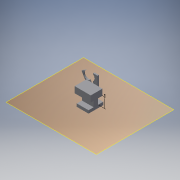
# Autodesk Inventor part: BSF_ShuttleFeeder
Saved by Autodesk Inventor 2018 (Build 220112000, 112)
## iProperties
Created: 2019-03-24
Part Number: BSF_ShuttleFeeder
Material: Generic
Document SubType Name: Modeling
Designer: simon
Density: 1 g/cm^3
Appearance: Default
Author: simon
Autodesk Inventor part; units mm, degrees
ref_plane "YZ Plane" through (0, 0, 0) normal (1, 0, 0) x (0, 1, 0)
ref_plane "XZ Plane" through (0, 0, 0) normal (0, 1, 0) x (-1, 0, 0)
ref_plane "Work Plane1" through (0, 0, 0) normal (0, 0, 1) x (1, 0, 0)
ref_plane "Work Plane2" through (-162, -84, 44) normal (0, 0, 1) x (1, 0, 0)
sketch "Sketch1" plane through (0, 0, 0) normal (0, 0, 1) x (1, 0, 0)
  line L0 (-280, 0) -> (-160, 0) projected
  line L1 (-280, 0) -> (-280, -40) projected
  line L2 (-162, -40) -> (-280, -40) projected
  line L3 (-118, -40) -> (-162, -40) projected
  line L4 (0, -40) -> (-118, -40) projected
  line L5 (0, 0) -> (0, -40) projected
  line L6 (-120, 0) -> (0, 0) projected
  line L7 (-120, 0) -> (-120, 160) projected
  line L8 (0, 160) -> (-120, 160) projected
  line L9 (0, 160) -> (0, 200) projected
  line L10 (-280, 200) -> (0, 200) projected
  line L11 (-280, 160) -> (-280, 200) projected
  line L12 (-160, 160) -> (-280, 160) projected
  line L13 (-160, 0) -> (-160, 160) projected
  line L14 (-160, 87.5) -> (-120, 87.5)
  line L15 (-120, 87.5) -> (-120, 72.5)
  line L16 (-120, 72.5) -> (-160, 72.5)
  line L17 (-160, 72.5) -> (-160, 87.5)
  line L18 (-160, 87.5) -> (-120, 72.5) construction
  line L19 (-120, 87.5) -> (-160, 72.5) construction
  point P0 (-140, 80)
  dimension "d0" = 40
  dimension "d1" = 15
  constraints: 12 end point, 2 midpoint, 2 parallel, 1 horizontal, 1 perpendicular
  measures "d0" distance of L15.end L16.end
  measures "d1" distance of L14.end L15.end
extrude "Extrusion1" add sketch "Sketch1" along normal up to surface (44 mm away) contours L13 L14 L7 L16
ref_plane "Work Plane3" through (0, 0, 0) normal (0, 0, 1) x (1, 0, 0)
sketch "Sketch2" plane through (0, 0, 0) normal (0, 0, 1) x (1, 0, 0)
  line L0 (-120, 87.5) -> (-120, 72.5) projected
  line L1 (-160, 87.5) -> (-120, 87.5) projected
  line L2 (-160, 72.5) -> (-160, 87.5) projected
  line L3 (-120, 72.5) -> (-160, 72.5) projected
  line L4 (-160, 105) -> (-120, 105)
  line L5 (-120, 105) -> (-120, 55)
  line L6 (-120, 55) -> (-160, 55)
  line L7 (-160, 55) -> (-160, 105)
  line L8 (-160, 105) -> (-120, 55) construction
  line L9 (-120, 105) -> (-160, 55) construction
  point P0 (0, 0)
  point P1 (-140, 80)
  dimension "d7" = 40
  dimension "d8" = 50
  constraints: 12 end point, 2 midpoint, 2 parallel, 1 horizontal, 1 perpendicular
  measures "d7" distance of L5.end L6.end
  measures "d8" distance of L4.end L5.end
extrude "Extrusion2" add sketch "Sketch2" along normal blind 10 contours L1 L7 L4 L5 | L5 L6 L7 L3
sketch "Sketch3" plane through (-160, 87.5, 44) normal (0, 1, 0) x (1, 0, 0)
  line L0 (0, 0) -> (55, 0)
  line L1 (55, 0) -> (55, -21)
  line L2 (55, -21) -> (0, -21)
  line L3 (0, -21) -> (0, 0)
  point P0 (160, 44)
  dimension "d11" = 55
  dimension "d12" = 21
  constraints: 8 end point, 2 parallel, 1 horizontal, 1 perpendicular
  measures "d11" distance of L1.end L2.end
  measures "d12" distance of L0.end L1.end
extrude "Extrusion3" add sketch "Sketch3" against normal blind 40
sketch "Sketch4" plane through (-160, 87.5, 10) normal (0, 1, 0) x (1, 0, 0)
  line L0 (40, 0) -> (0, 0) projected
  line L1 (0, 0) -> (0, -55) projected
  line L2 (55, -55) -> (0, -55) projected
  line L3 (55, -34) -> (55, -55) projected
  line L4 (40, -34) -> (55, -34) projected
  line L5 (40, 0) -> (40, -34) projected
  line L6 (55, -55) -> (0, -55) projected
  line L7 (55, -34) -> (0, -34)
  line L8 (0, -34) -> (0, -55)
  line L9 (0, -55) -> (55, -55)
  line L10 (55, -55) -> (55, -34)
  line L11 (0, -44.5) -> (15, -44.5)
  line L12 (0, -44.5) -> (15, -44.5) construction
  circle A0 centre (15, -44.5) radius 4
  point P0 (160, 10)
  dimension "d15" = 15
  dimension "d16" = 0
  dimension "d17" = 8
  constraints: 12 end point, 3 horizontal, 2 parallel, 1 centre point, 1 coincident, 1 collinear, 1 midpoint, 1 perpendicular
  measures "d15" distance of L11.start L11.end
  measures "d16" distance between parallel lines of L11 L12
  measures "d17" diameter of A0
extrude "Extrusion4" add sketch "Sketch4" along normal blind 8 contours A0
sketch "Sketch5" plane through (-160, 87.5, 10) normal (0, 1, 0) x (1, 0, 0)
  circle A0 centre (15, -44.5) radius 4 projected
  line L0 (40, 0) -> (0, 0) projected
  line L1 (0, 0) -> (0, -55) projected
  line L2 (55, -55) -> (0, -55) projected
  line L3 (55, -34) -> (55, -55) projected
  line L4 (40, -34) -> (55, -34) projected
  line L5 (40, 0) -> (40, -34) projected
  circle A1 centre (15, -44.5) radius 4 projected
  line L6 (15, -44.5) -> (28, -44.5)
  line L7 (15, -44.5) -> (28, -44.5) construction
  line L8 (15, -44.5) -> (2, -44.5)
  line L9 (15, -44.5) -> (28, -44.5) construction
  line L10 (28, -44.5) -> (38, -44.5)
  line L11 (38, -44.5) -> (38, -84.5)
  line L12 (38, -84.5) -> (28, -84.5)
  line L13 (28, -84.5) -> (28, -44.5)
  line L14 (28, -44.5) -> (23, -44.5)
  line L15 (23, -44.5) -> (23, -84.5)
  line L16 (23, -84.5) -> (28, -84.5)
  line L17 (28, -84.5) -> (28, -44.5)
  line L18 (3.5452, -38.0217) -> (16.5356, -45.5217)
  line L19 (16.5356, -45.5217) -> (-3.4644, -80.1628)
  line L20 (-3.4644, -80.1628) -> (-16.4548, -72.6628)
  line L21 (-16.4548, -72.6628) -> (3.5452, -38.0217)
  line L22 (3.5452, -38.0217) -> (8.5452, -29.3615)
  line L23 (8.5452, -29.3615) -> (21.5356, -36.8615)
  line L24 (21.5356, -36.8615) -> (16.5356, -45.5217)
  point P0 (160, 10)
  dimension "d20" = 13
  dimension "d21" = 0
  dimension "d22" = 13
  dimension "d23" = 180
  dimension "d24" = 10
  dimension "d25" = 40
  dimension "d26" = 5
  dimension "d27" = 15
  dimension "d28" = 40
  dimension "d31" = 10
  constraints: 38 end point, 6 horizontal, 6 parallel, 4 perpendicular, 3 collinear, 1 point on line
  measures "d20" distance of L6.start L6.end
  measures "d21" distance between parallel lines of L6 L7
  measures "d22" distance of L6.start L8.end
  measures "d23" angle of L8 L9
  measures "d24" distance of L11.end L12.end
  measures "d25" distance of L10.end L11.end
  measures "d26" distance of L16.end L15.end
  measures "d27" distance of L19.end L20.end
  measures "d28" distance of L18.end L19.end
  measures "d31" distance of L18.start L22.end
extrude "Extrusion5" add sketch "Sketch5" along normal blind 5 contours L24 L6 L8 L18 A0 | A0 L18 L22 L23 L24 | L19 L2 L1 L21 L18 A0 | A0 L8 L18 L19 | L6 L13 L2 L15 | L24 L18 L8 L6 | L18 L8 A0 | L19 L20 L21 L1 L2 | L10 L11 L2 L13 | L2 L13 L16 L15 | L2 L11 L12 L13
sketch "Sketch6" plane through (-160, 92.5, 10) normal (0, 1, 0) x (1, 0, 0)
  line L0 (23, -84.5) -> (38, -84.5) projected
  line L1 (38, -84.5) -> (38, -44.5) projected
  line L2 (38, -44.5) -> (23, -44.5) projected
  line L3 (23, -44.5) -> (23, -84.5) projected
  arc A0 (18.3698, -42.3448) -> (14.8185, -48.4959) centre (15, -44.5) ccw projected
  line L4 (18.3698, -42.3448) -> (21.5356, -36.8615) projected
  line L5 (21.5356, -36.8615) -> (8.5452, -29.3615) projected
  line L6 (8.5452, -29.3615) -> (-16.4548, -72.6628) projected
  line L7 (-16.4548, -72.6628) -> (-3.4644, -80.1628) projected
  line L8 (-3.4644, -80.1628) -> (14.8185, -48.4959) projected
  circle A1 centre (15, -44.5) radius 4 projected
  line L9 (15, -44.5) -> (15, -71.5)
  circle A2 centre (15, -71.5) radius 13
  line L10 (15, -44.5) -> (3.1255, -68.7486)
  circle A3 centre (3.1255, -68.7486) radius 13
  point P0 (160, 10)
  dimension "d32" = 27
  dimension "d33" = 26
  dimension "d34" = 27
  dimension "d35" = 26
  constraints: 4 end point, 2 centre point, 2 coincident, 1 point on line, 1 vertical
  measures "d32" distance of L9.start L9.end
  measures "d33" diameter of A2
  measures "d34" distance of L9.start L10.end
  measures "d35" diameter of A3
extrude "Extrusion6" cut sketch "Sketch6" against normal blind 5 contours A2 A3 L9 L3 | L3 A2 | A3 L8 A2 | A2 L8 A3 | L9 A3 A2 | A2 L10 L8 | L8 A3 L10 A2 | A2 L8 A3 | L10 A2 L8 | L10 A3 L8 A2
equation "\"d34\" = d32"
equation "\"d35\" = d33"
body "Solid1"
